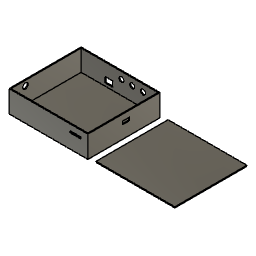
boxcts (Autodesk Fusion 360 design; units mm, degrees)
Autodesk Fusion 360 part; units mm, degrees
sketch "Sketch1" plane through (0, 0, 0) normal (0, 0, 1) x (1, 0, 0)
  line L0 (-49.2609, 64.2986) -> (52.9391, 64.2986)
  line L1 (52.9391, 64.2986) -> (52.9391, -29.1014)
  line L2 (52.9391, -29.1014) -> (-49.2609, -29.1014)
  line L3 (-49.2609, -29.1014) -> (-49.2609, 64.2986)
  dimension "d1" = 102.2
  dimension "d2" = 93.4
  constraint horizontal L0
  constraint vertical L1
  constraint horizontal L2
  constraint vertical L3
  measures "d1" distance of L0.start L0.end
  measures "d2" distance of L0.start L2.end
extrude "Extrude1" add sketch "Sketch1" along normal blind 1.2 makes body 1
sketch "Sketch2" plane through (0, 0, 1.2) normal (0, 0, 1) x (-1, 0, 0)
  line L0 (49.2609, 29.1014) -> (-52.9391, 29.1014)
  line L1 (-52.9391, 29.1014) -> (-52.9391, -64.2986)
  line L2 (-52.9391, -64.2986) -> (49.2609, -64.2986)
  line L3 (49.2609, -64.2986) -> (49.2609, 29.1014)
  line L4 (49.2609, -64.2986) -> (-52.9391, -64.2986)
  line L5 (-52.9391, -64.2986) -> (-52.9391, -63.0986)
  line L6 (-52.9391, -63.0986) -> (49.2609, -63.0986)
  line L7 (49.2609, -63.0986) -> (49.2609, -64.2986)
  line L8 (49.2609, -64.2986) -> (48.0609, -64.2986)
  line L9 (48.0609, -64.2986) -> (48.0609, 29.1014)
  line L10 (48.0609, 29.1014) -> (49.2609, 29.1014)
  line L11 (49.2609, 29.1014) -> (49.2609, -64.2986)
  line L12 (-52.9391, -64.2986) -> (-51.7391, -64.2986)
  line L13 (-51.7391, -64.2986) -> (-51.7391, 29.1014)
  line L14 (-51.7391, 29.1014) -> (-52.9391, 29.1014)
  line L15 (-52.9391, 29.1014) -> (-52.9391, -64.2986)
  line L16 (49.2609, 29.1014) -> (-52.9391, 29.1014)
  line L17 (-52.9391, 29.1014) -> (-52.9391, 27.9014)
  line L18 (-52.9391, 27.9014) -> (49.2609, 27.9014)
  line L19 (49.2609, 27.9014) -> (49.2609, 29.1014)
  dimension "d5" = 1.2
  dimension "d6" = 1.2
  dimension "d7" = 1.2
  dimension "d8" = 1.2
  constraint horizontal L4
  constraint vertical L5
  constraint horizontal L6
  constraint vertical L7
  constraint coincident L1 L5.end
  constraint coincident L2.end L3.start
  constraint horizontal L8
  constraint vertical L9
  constraint horizontal L10
  constraint vertical L11
  constraint horizontal L12
  constraint vertical L13
  constraint horizontal L14
  constraint vertical L15
  constraint horizontal L16
  constraint vertical L17
  constraint horizontal L18
  constraint vertical L19
  constraint coincident L15 L17.end
  constraint collinear L0 L16
  constraint collinear L14 L16
  measures "d5" distance of L2.end L6.end
  measures "d6" distance of L2.end L8.end
  measures "d7" distance of L1.end L12.end
  measures "d8" distance of L0.start L18.end
extrude "Extrude2" add sketch "Sketch2" along normal blind 27.2 contours L0 L3 L9 L10 L11 L16 L18 L19 | L0 L9 L13 L16 L18 | L3 L6 L9 L11 L18 | L0 L1 L13 L14 L15 L16 L17 L18 | L2 L3 L4 L6 L7 L8 L9 L11 | L1 L6 L13 L15 L18 | L2 L4 L6 L9 L13 | L1 L2 L4 L5 L6 L12 L13 L15 bodies 1
sketch "Sketch3" plane through (0, 0, 1.2) normal (0, 0, 1) x (-1, 0, 0)
  line L0 (48.0609, 27.9014) -> (-51.7391, 27.9014)
  line L1 (-51.7391, 27.9014) -> (-51.7391, -63.0986)
  line L2 (-51.7391, -63.0986) -> (48.0609, -63.0986)
  line L3 (48.0609, -63.0986) -> (48.0609, 27.9014)
  line L4 (-165, -65) -> (-62.8, -65)
  line L5 (-62.8, -65) -> (-62.8, 28.4)
  line L6 (-62.8, 28.4) -> (-165, 28.4)
  line L7 (-165, 28.4) -> (-165, -65)
  dimension "d11" = 102.2
  dimension "d12" = 93.4
  constraint horizontal L4
  constraint vertical L5
  constraint horizontal L6
  constraint vertical L7
  measures "d11" distance of L4.start L4.end
  measures "d12" distance of L4.start L6.end
extrude "Extrude3" add sketch "Sketch3" along normal blind 1.2 separate body contours L4 L5 L6 L7 makes body 2
sketch "Sketch4" plane through (0, -29.1014, 0) normal (0, -1, 0) x (1, 0, 0)
  line L0 (-49.2609, 0) -> (52.9391, 0)
  line L1 (52.9391, 0) -> (52.9391, 28.4)
  line L2 (52.9391, 28.4) -> (-49.2609, 28.4)
  line L3 (-49.2609, 28.4) -> (-49.2609, 0)
  line L4 (29.7391, 20.6) -> (43.7391, 20.6)
  line L5 (43.7391, 20.6) -> (43.7391, 18.4)
  line L6 (43.7391, 18.4) -> (29.7391, 18.4)
  line L7 (29.7391, 18.4) -> (29.7391, 20.6)
  dimension "d15" = 18.4
  dimension "d16" = 9.2
  dimension "d17" = 14
  dimension "d18" = 2.2
  constraint horizontal L4
  constraint vertical L5
  constraint horizontal L6
  constraint vertical L7
  measures "d15" distance of L0 L6
  measures "d16" distance of L1 L5
  measures "d17" distance of L4.start L4.end
  measures "d18" distance of L4.start L6.end
extrude "Extrude4" cut sketch "Sketch4" against normal blind 4 contours L4 L5 L6 L7 bodies 1
sketch "Sketch5" plane through (0, 64.2986, 0) normal (0, 1, 0) x (-1, 0, 0)
  line L0 (-52.9391, 0) -> (49.2609, 0)
  line L1 (49.2609, 0) -> (49.2609, 28.4)
  line L2 (49.2609, 28.4) -> (-52.9391, 28.4)
  line L3 (-52.9391, 28.4) -> (-52.9391, 0)
  circle A0 centre (-32.2391, 19.2) radius 3.2
  line L4 (-51.7391, 1.2) -> (-51.7391, 28.4)
  line L5 (7.0609, 12) -> (17.0609, 12)
  line L6 (17.0609, 12) -> (17.0609, 5)
  line L7 (17.0609, 5) -> (7.0609, 5)
  line L8 (7.0609, 5) -> (7.0609, 12)
  circle A1 centre (-18.2391, 19.2) radius 3.2
  circle A2 centre (-4.2391, 19.2) radius 3.2
  dimension "d21" = 6.4
  dimension "d22" = 19.2
  dimension "d26" = 10
  dimension "d27" = 7
  dimension "d28" = 32.2
  dimension "d30" = 5
  dimension "d44" = 20.7
  dimension "d45" = 6.4
  dimension "d46" = 6.4
  constraint horizontal L5
  constraint vertical L6
  constraint horizontal L7
  constraint vertical L8
  measures "d21" diameter of A0
  measures "d22" distance of L0 A0.centre
  measures "d26" distance of L5.start L5.end
  measures "d27" distance of L5.start L7.end
  measures "d28" distance of L1 L6
  measures "d30" distance of L0 L7
  measures "d44" distance of L3 A0.centre
  measures "d45" diameter of A1
  measures "d46" diameter of A2
extrude "Extrude5" cut sketch "Sketch5" against normal blind 4 contours A0 | L5 L6 L7 L8 | A1 | A2 bodies 1
sketch "Sketch6" plane through (52.9391, 0, 0) normal (1, 0, 0) x (0, 1, 0)
  line L0 (-29.1014, 0) -> (64.2986, 0)
  line L1 (64.2986, 0) -> (64.2986, 28.4)
  line L2 (64.2986, 28.4) -> (-29.1014, 28.4)
  line L3 (-29.1014, 28.4) -> (-29.1014, 0)
  line L4 (16.0986, 20.5) -> (25.0986, 20.5)
  line L5 (25.0986, 20.5) -> (25.0986, 16.5)
  line L6 (25.0986, 16.5) -> (16.0986, 16.5)
  line L7 (16.0986, 16.5) -> (16.0986, 20.5)
  dimension "d33" = 4
  dimension "d34" = 9
  dimension "d35" = 16.5
  dimension "d36" = 39.2
  constraint horizontal L4
  constraint vertical L5
  constraint horizontal L6
  constraint vertical L7
  measures "d33" distance of L4.end L5.end
  measures "d34" distance of L4.start L4.end
  measures "d35" distance of L0 L6
  measures "d36" distance of L1 L5
extrude "Extrude6" cut sketch "Sketch6" against normal blind 2 contours L4 L5 L6 L7 bodies 1
sketch "Sketch7" plane through (-49.2609, 0, 0) normal (-1, 0, 0) x (0, -1, 0)
  line L0 (-64.2986, 0) -> (29.1014, 0)
  line L1 (29.1014, 0) -> (29.1014, 28.4)
  line L2 (29.1014, 28.4) -> (-64.2986, 28.4)
  line L3 (-64.2986, 28.4) -> (-64.2986, 0)
  circle A0 centre (9.1014, 22) radius 3.5
  dimension "d39" = 7
  dimension "d40" = 20
  dimension "d41" = 22
  measures "d39" diameter of A0
  measures "d40" distance of L1 A0.centre
  measures "d41" distance of L0 A0.centre
extrude "Extrude7" cut sketch "Sketch7" against normal blind 3 contours A0 bodies 1
equation "d1 = 97.8 mm + 2.4 mm + 2 mm"
equation "d2 = 89 mm + 2.4 mm + 2 mm"
equation "d9 = 30 mm - 2.8 mm"
equation "d15 = 13 mm + 1.4 mm + 4 mm"
equation "d16 = 7 mm + 1 mm + 1.2 mm"
equation "d22 = 14 mm + 4 mm + 1.2 mm"
equation "d28 = 30 mm + 1 mm + 1.2 mm"
equation "d30 = 3.8 mm + 1.2 mm"
equation "d35 = 11.3 mm + 4 mm + 1.2 mm"
equation "d36 = 37 mm + 1.2 mm + 1 mm"
equation "d44 = 18.5 mm + 1 mm + 1.2 mm"
